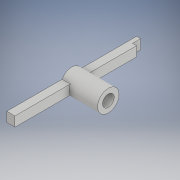
# Autodesk Inventor part: LiftMotorHousingOne
Saved by Autodesk Inventor 2019 (Build 230136000, 136)
## iProperties
Created: 2018-09-19
Part Number: LiftMotorHousingOne
Material: Generic
Document SubType Name: Modeling
Designer: hale985
Density: 1 g/cm^3
Appearance: Default
Author: hale985
Autodesk Inventor part; units mm, degrees
ref_plane "YZ Plane" through (0, 0, 0) normal (1, 0, 0) x (0, 1, 0)
ref_plane "XZ Plane" through (0, 0, 0) normal (0, 1, 0) x (-1, 0, 0)
ref_plane "XY Plane" through (0, 0, 0) normal (0, 0, 1) x (1, 0, 0)
sketch "Sketch1" plane through (0, 0, 0) normal (1, 0, 0) x (0, 1, 0)
  circle A0 centre (0, 0) radius 4.572
  circle A1 centre (0, 0) radius 8.382
  dimension "d0" = 9.144
  dimension "d1" = 3.81
  constraints: 2 centre point, 1 coincident
  measures "d0" diameter of A0
  measures "d1" radial gap between concentric circles of A0 A1
extrude "Extrusion1" add sketch "Sketch1" along normal blind 19.812
sketch "Sketch2" plane through (0, 0, 0) normal (-1, 0, 0) x (0, 0, 1)
  circle A0 centre (0, 0) radius 8.382
  circle A1 centre (0, 0) radius 7.747
  circle A2 centre (0, 0) radius 8.382 projected
  dimension "d42" = 0
  constraints: 2 centre point, 2 coincident
  measures "d42" radial gap between concentric circles of A2 A0
extrude "Extrusion2" add sketch "Sketch2" along normal blind 2.54 contours A0 | A1
sketch "Sketch10" plane through (0, 0, 0) normal (1, 0, 0) x (0, 0, -1)
  circle A0 centre (0, 0) radius 1.4542
  line L0 (-4.572, 1.4542) -> (4.572, 1.4542)
  line L1 (4.572, 1.4542) -> (4.572, -1.4542)
  line L2 (4.572, -1.4542) -> (-4.572, -1.4542)
  line L3 (-4.572, -1.4542) -> (-4.572, 1.4542)
  circle A1 centre (0, 0) radius 4.572 projected
  dimension "d43" = 0
  dimension "d44" = 0
  constraints: 8 end point, 2 parallel, 1 centre point, 1 coincident, 1 horizontal, 1 perpendicular
  measures "d43" distance edge to line of A1 L1
  measures "d44" distance edge to line of A1 L3
extrude "Extrusion7" cut sketch "Sketch10" against normal blind 22.225 contours A0 | A0 L0 A1 L2 | A0 L2 A1 L0 | A1 L3 L0 | L0 L1 A1 | A1 L1 L2 | L2 L3 A1
sketch "Sketch24" plane through (-2.54, 0, 0) normal (-1, 0, 0) x (0, 0, 1)
  line L0 (50.8, -3.81) -> (-50.8, -3.81)
  line L1 (-50.8, -3.81) -> (-50.8, 3.81)
  line L2 (-50.8, 3.81) -> (50.8, 3.81)
  line L3 (50.8, 3.81) -> (50.8, -3.81)
  line L4 (4.572, 1.4542) -> (4.572, -1.4542) projected
  line L5 (4.572, -1.4542) -> (-4.572, -1.4542) projected
  line L6 (-4.572, -1.4542) -> (-4.572, 1.4542) projected
  line L7 (-4.572, 1.4542) -> (4.572, 1.4542) projected
  circle A0 centre (0, 0) radius 8.382 projected
  dimension "d90" = 101.6
  dimension "d91" = 50.8
  dimension "d92" = 3.81
  dimension "d93" = 3.81
  constraints: 8 end point, 2 parallel, 1 horizontal, 1 perpendicular
  measures "d90" distance of L1.end L2.end
  measures "d91" distance from line of point (0, 0) L1
  measures "d92" distance from line of L0 point (0, 0)
  measures "d93" distance from line of L2 point (0, 0)
extrude "Extrusion18" add sketch "Sketch24" along normal blind 6.35 contours L0 A0 L2 L3 | L0 A0 L2 | L0 L1 L2 A0
sketch "Sketch25" plane through (-2.54, 0, 0) normal (-1, 0, 0) x (0, 0, 1)
  line L0 (-7.466, 3.81) -> (7.466, 3.81) projected
  arc A0 (7.466, 3.81) -> (-7.466, 3.81) centre (0, 0) ccw projected
  line L1 (7.466, -3.81) -> (-7.466, -3.81) projected
  arc A1 (-7.466, -3.81) -> (7.466, -3.81) centre (0, 0) ccw projected
extrude "Extrusion19" add sketch "Sketch25" along normal blind 6.35
sketch "Sketch26" plane through (-2.54, -3.81, 7.466) normal (0, -1, 0) x (1, 0, 0)
  line L0 (0, 0) -> (0, 43.334) projected
  line L1 (0, 43.334) -> (-3.175, 43.334)
  line L2 (-3.175, 43.334) -> (-3.175, 36.984)
  line L3 (-3.175, 36.984) -> (0, 36.984)
  line L4 (0, 36.984) -> (0, 43.334)
  point P0 (2.54, -7.466)
  dimension "d98" = 3.175
  dimension "d99" = 6.35
  constraints: 8 end point, 2 parallel, 1 horizontal, 1 perpendicular
  measures "d98" distance of L3.end L2.end
  measures "d99" distance of L2.end L1.end
extrude "Extrusion20" cut sketch "Sketch26" against normal blind 25.4
body "Solid1"
